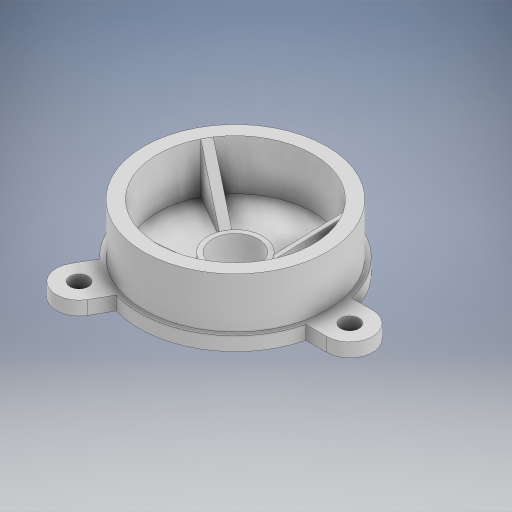
# Autodesk Inventor part: CE-2.1.4-01
Saved by Autodesk Inventor 2024 (Build 280153000, 153)
## iProperties
Created: 2024-01-31
Part Number: CE-2.1.4-01
Material: Generic
Document SubType Name: Modeling
Designer: Alex
Density: 1 g/cm^3
Appearance: Default
Author: Alex
Autodesk Inventor part; units mm, degrees
ref_plane "YZ Plane" through (0, 0, 0) normal (1, 0, 0) x (0, 1, 0)
ref_plane "XZ Plane" through (0, 0, 0) normal (0, 1, 0) x (-1, 0, 0)
ref_plane "XY Plane" through (0, 0, 0) normal (0, 0, 1) x (1, 0, 0)
sketch "Sketch1" plane through (0, 0, 0) normal (0, 1, 0) x (-1, 0, 0)
  circle A0 centre (0, 0) radius 25 construction
  circle A1 centre (0, 0) radius 21
  circle A2 centre (0, 0) radius 20
  circle A3 centre (0, 0) radius 17
  circle A4 centre (0, 0) radius 10
  circle A5 centre (0, 0) radius 6
  circle A6 centre (0, 0) radius 5
  arc A7 (-25, 5) -> (-25, -5) centre (-25, 0) ccw
  circle A8 centre (-25, 0) radius 2
  line L0 (-25, 5) -> (-20.3961, 5)
  line L1 (-25, -5) -> (-20.3961, -5)
  line L2 (0, 0) -> (-25, 0) construction
  dimension "d0" = 50
  dimension "d1" = 42
  dimension "d2" = 40
  dimension "d3" = 34
  dimension "d4" = 20
  dimension "d5" = 12
  dimension "d6" = 10
  dimension "d7" = 4
  dimension "d8" = 5
  constraints: 8 centre point, 8 coincident, 6 end point, 4 point on circle, 3 horizontal, 2 tangent, 1 horizontal alignment, 2 other
  measures "d1" diameter of A1
  measures "d2" diameter of A2
  measures "d3" diameter of A3
  measures "d4" diameter of A4
  measures "d5" diameter of A5
  measures "d6" diameter of A6
  measures "d7" diameter of A8
  measures "d8" radius of A7
extrude "Extrusion1" add sketch "Sketch1" along normal blind 3 contours A1 | A2 | A3 | A4 | A5
extrude "Extrusion2" add sketch "Sketch1" against normal blind 3 contours A4 | A5
extrude "Extrusion3" add sketch "Sketch1" along normal blind 14 contours A2
extrude "Extrusion4" add sketch "Sketch1" along normal blind 4 contours A5
sketch "Sketch2" plane through (0, 0, 0) normal (0, 1, 0) x (-1, 0, 0)
  arc A0 (-25, 5) -> (-25, -5) centre (-25, 0) ccw projected
  line L0 (-25, 5) -> (-20.3961, 5) projected
  line L1 (-25, -5) -> (-20.3961, -5) projected
  circle A1 centre (-25, 0) radius 2 projected
  circle A2 centre (0, 0) radius 21 construction
  arc A3 (-20.3961, 5) -> (-20.3961, -5) centre (0, 0) ccw
  constraints: 2 point on circle, 1 centre point, 1 concentric
extrude "Extrusion5" add sketch "Sketch2" along normal up to surface (3 mm away)
pattern_circular "Circular Pattern1" count 3 over 360 about axis through (0, -10, 0) along (0, 1, 0) of "Extrusion5"
sketch "Sketch3" plane through (0, 0, 0) normal (1, 0, 0) x (0, 1, 0)
  line L0 (14, 17) -> (3, 17) construction
  line L1 (14, -17) -> (3, -17) construction
  line L2 (3, -17) -> (3, 17) construction
  line L3 (3, 6) -> (4, 6) construction
  line L4 (4, -6) -> (4, 6) construction
  line L5 (3, -6) -> (4, -6) construction
  line L6 (3, -20) -> (14, -20) construction
  line L7 (14, -20) -> (14, 20) construction
  line L8 (3, 20) -> (14, 20) construction
  line L9 (3, 5) -> (3, 21) construction
  line L10 (3, -21) -> (3, -5) construction
  line L11 (0, -21) -> (3, -21) construction
  line L12 (0, 21) -> (3, 21) construction
  line L13 (0, 5) -> (0, 21) construction
  line L14 (0, -10) -> (0, 10) construction
  line L15 (0, -15.1635) -> (0, 15.1635) construction
  line L16 (0, -19.1506) -> (0, -15.1635) construction
  line L17 (0, -21) -> (0, -5) construction
  line L18 (0, -21) -> (3, -21) construction
  line L19 (14, 17) -> (4, 6)
  line L20 (14, 17) -> (4, 17)
  point P0 (0, 0)
  point P1 (3, 20.1635)
  point P2 (3, -20.1635)
  point P3 (0, 20.1635)
  point P4 (0, -20.1635)
  constraints: 4 end point, 1 collinear
extrude "Rib1" add sketch "Sketch3" along normal mid plane 2 rib yes fills toward (8.963, 11.5336) open curves L19 L20
pattern_circular "Circular Pattern2" count 3 over 360 about axis through (0, -10, 0) along (0, 1, 0) of "Rib1"
body "Solid1"
